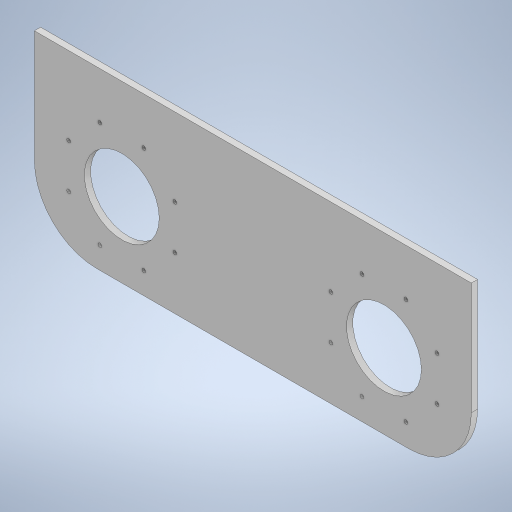
# Autodesk Inventor part: legparts_09(six)
Saved by Autodesk Inventor 2024.3 (Build 283343000, 343)
## iProperties
Created: 2025-01-05
Part Number: legparts_09(six)
Material: 一般
Document SubType Name: Modeling
Designer: 佐藤智貴
Density: 1 g/cm^3
Appearance: 既定
Author: 佐藤智貴
Autodesk Inventor part; units mm, degrees
ref_plane "YZ Plane" through (0, 0, 0) normal (1, 0, 0) x (0, 1, 0)
ref_plane "XZ Plane" through (0, 0, 0) normal (0, 1, 0) x (-1, 0, 0)
ref_plane "XY Plane" through (0, 0, 0) normal (0, 0, 1) x (1, 0, 0)
sketch "スケッチ1" plane through (0, 0, 0) normal (0, 0, 1) x (1, 0, 0)
  line L0 (0, 0) -> (350, 0)
  line L1 (350, 0) -> (350, 140)
  line L2 (350, 140) -> (0, 140)
  circle A0 centre (70, 60) radius 46
  circle A1 centre (280, 60) radius 46
  line L3 (0, 140) -> (0, 0)
  line L4 (70, 60) -> (70, 156.3161)
  line L5 (280, 60) -> (280, 147.5689)
  line L6 (70, 60) -> (45.2011, 119.8698)
  line L7 (280, 60) -> (258.2896, 112.4136)
  circle A2 centre (52.3966, 102.4985) radius 1.5
  circle A3 centre (262.3966, 102.4985) radius 1.5
  circle A4 centre (27.5015, 77.6034) radius 1.5
  circle A5 centre (27.5015, 42.3966) radius 1.5
  circle A6 centre (52.3966, 17.5015) radius 1.5
  circle A7 centre (87.6034, 17.5015) radius 1.5
  circle A8 centre (112.4985, 42.3966) radius 1.5
  circle A9 centre (112.4985, 77.6034) radius 1.5
  circle A10 centre (87.6034, 102.4985) radius 1.5
  circle A11 centre (237.5015, 77.6034) radius 1.5
  circle A12 centre (237.5015, 42.3966) radius 1.5
  circle A13 centre (262.3966, 17.5015) radius 1.5
  circle A14 centre (297.6034, 17.5015) radius 1.5
  circle A15 centre (322.4985, 42.3966) radius 1.5
  circle A16 centre (322.4985, 77.6034) radius 1.5
  circle A17 centre (297.6034, 102.4985) radius 1.5
  circle A18 centre (70, 60) radius 30
  circle A19 centre (280, 60) radius 30
  dimension "d5" = 92
  dimension "d6" = 92
  dimension "d0" = 350
  dimension "d1" = 140
  dimension "d2" = 60
  dimension "d3" = 60
  dimension "d9" = 70
  dimension "d10" = 70
  dimension "d11" = 22.5
  dimension "d12" = 22.5
  dimension "d13" = 3
  dimension "d14" = 3
  dimension "d17" = 360
  dimension "d21" = 360
  dimension "d23" = 60
  dimension "d24" = 60
  constraints: 18 centre point, 16 end point, 3 vertical, 2 point on line, 1 coincident, 1 horizontal, 1 parallel, 1 perpendicular, 40 other
  measures "d0" distance of L1.end L2.end
  measures "d1" distance of L0.end L1.end
  measures "d2" distance from line of L0 L4.start
  measures "d3" distance from line of L0 L5.start
  measures "d9" distance from line of L3 L4.start
  measures "d10" distance from line of L1 L5.start
  measures "d11" angle of L4 L6
  measures "d12" angle of L5 L7
  measures "d13" diameter of A2
  measures "d14" diameter of A3
  measures "d23" diameter of A18
  measures "d24" diameter of A19
extrude "押し出し1" add sketch "スケッチ1" along normal blind 5 contours A1 A17 A16 A15 A14 A13 A12 A11 A3 L7 A19 L5 | L5 A19 L7 A3 A1 | A0 A10 A9 A8 A7 A6 A5 A4 A2 L6 A18 L4 | L4 A18 L6 A2 A0 | L3 L2 L1 L0
fillet "フィレット2" radius 50 2 edges at (350, 0, 2.5) (0, 0, 2.5)
equation "\"d6\" = d5"
equation "\"d2\" = d3"
equation "\"d10\" = d9"
